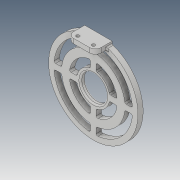
# Autodesk Inventor part: backSideThrusterCover
Saved by Autodesk Inventor 2018 (Build 220112000, 112)
## iProperties
Created: 2020-02-23
Part Number: backSideThrusterCover
Material: Generic
Document SubType Name: Modeling
Designer: anirudh
Density: 1 g/cm^3
Appearance: Default
Author: anirudh
Autodesk Inventor part; units mm, degrees
ref_plane "YZ Plane" through (0, 0, 0) normal (1, 0, 0) x (0, 1, 0)
ref_plane "XZ Plane" through (0, 0, 0) normal (0, 1, 0) x (-1, 0, 0)
ref_plane "XY Plane" through (0, 0, 0) normal (0, 0, 1) x (1, 0, 0)
sketch "Sketch1" plane through (0, 0, 0) normal (0, 0, 1) x (1, 0, 0)
  line L0 (3, 0) -> (-3, 0)
  line L1 (0, 0) -> (13.85, 0)
  line L2 (14.85, -3.0647) -> (14.85, -1)
  line L3 (14.85, -3.0647) -> (14.85, -1)
  line L4 (0, 0) -> (-13.85, 0)
  line L5 (13.85, 0) -> (-13.85, 0)
  line L6 (-14.85, -3.0647) -> (-14.85, -1)
  line L7 (-14.85, -3.0647) -> (-14.85, -1)
  arc A0 (47.8846, -42.8653) -> (14.85, -3.0647) centre (0, -49) ccw
  arc A1 (-14.85, -3.0647) -> (14.85, -3.0647) centre (0, -49) ccw
  circle A2 centre (0, -49) radius 13.97
  arc A3 (3.175, -66.4942) -> (17.4942, -52.175) centre (0, -49) ccw
  arc A4 (-17.4942, -52.175) -> (-3.175, -66.4942) centre (0, -49) ccw
  arc A5 (17.4942, -45.825) -> (3.175, -31.5058) centre (0, -49) ccw
  arc A6 (-3.175, -31.5058) -> (-17.4942, -45.825) centre (0, -49) ccw
  line L8 (-17.4942, -52.175) -> (-25.8407, -52.175)
  line L9 (-34.1427, -52.175) -> (-42.4264, -52.175)
  line L10 (-3.175, -66.4942) -> (-3.175, -74.8407)
  line L11 (-3.175, -83.1427) -> (-3.175, -91.4264)
  arc A7 (-25.8407, -52.175) -> (-3.175, -74.8407) centre (0, -49) ccw
  line L12 (3.175, -66.4942) -> (3.175, -74.8407)
  line L13 (3.175, -83.1427) -> (3.175, -91.4264)
  line L14 (17.4942, -52.175) -> (25.8407, -52.175)
  line L15 (34.1427, -52.175) -> (42.4264, -52.175)
  arc A8 (3.175, -74.8407) -> (25.8407, -52.175) centre (0, -49) ccw
  line L16 (17.4942, -45.825) -> (25.8407, -45.825)
  line L17 (34.1427, -45.825) -> (42.4264, -45.825)
  line L18 (3.175, -31.5058) -> (3.175, -23.1593)
  line L19 (3.175, -14.8573) -> (3.175, -6.5736)
  arc A9 (25.8407, -45.825) -> (3.175, -23.1593) centre (0, -49) ccw
  arc A10 (-3.175, -23.1593) -> (-25.8407, -45.825) centre (0, -49) ccw
  line L20 (-3.175, -31.5058) -> (-3.175, -23.1593)
  line L21 (-3.175, -14.8573) -> (-3.175, -6.5736)
  line L22 (-17.4942, -45.825) -> (-25.8407, -45.825)
  line L23 (-34.1427, -45.825) -> (-42.4264, -45.825)
  arc A11 (-42.4264, -52.175) -> (-3.175, -91.4264) centre (0, -49) ccw
  arc A12 (-34.1427, -52.175) -> (-3.175, -83.1427) centre (0, -49) ccw
  arc A13 (3.175, -91.4264) -> (42.4264, -52.175) centre (0, -49) ccw
  arc A14 (3.175, -83.1427) -> (34.1427, -52.175) centre (0, -49) ccw
  arc A15 (34.1427, -45.825) -> (3.175, -14.8573) centre (0, -49) ccw
  arc A16 (-3.175, -14.8573) -> (-34.1427, -45.825) centre (0, -49) ccw
  arc A17 (42.4264, -45.825) -> (3.175, -6.5736) centre (0, -49) ccw
  arc A18 (-3.175, -6.5736) -> (-42.4264, -45.825) centre (0, -49) ccw
  line L24 (-14.85, -1) -> (-14.85, 0)
  line L25 (-14.85, 0) -> (-13.85, 0)
  line L26 (14.85, -1) -> (14.85, 0)
  line L27 (14.85, 0) -> (13.85, 0)
  point P0 (0, 0)
  point P1 (0, -49)
  point P2 (-16.85, -4.0995)
  constraints: 57 end point, 36 point on circle, 19 centre point, 8 parallel, 6 coincident, 6 perpendicular, 5 vertical, 2 horizontal, 1 collinear, 1 midpoint
extrude "Extrusion1" add sketch "Sketch1" along normal blind 5.588
fillet "Fillet1" radius 1.5875 34 edges at (14.85, -3.0647, 2.794) (-14.85, -3.0647, 2.794) (3.175, -6.5736, 2.794) (3.175, -14.8573, 2.794) (3.175, -23.1593, 2.794) (3.175, -31.5058, 2.794) (17.4942, -45.825, 2.794) (25.8407, -45.825, 2.794) (34.1427, -45.825, 2.794) (42.4264, -45.825, 2.794) (-3.175, -66.4942, 2.794) (-3.175, -74.8407, 2.794) (-3.175, -83.1427, 2.794) (-3.175, -91.4264, 2.794) (3.175, -91.4264, 2.794) (3.175, -83.1427, 2.794) (3.175, -74.8407, 2.794) (3.175, -66.4942, 2.794) (17.4942, -52.175, 2.794) (25.8407, -52.175, 2.794) (34.1427, -52.175, 2.794) (42.4264, -52.175, 2.794) (-42.4264, -52.175, 2.794) (-34.1427, -52.175, 2.794) (-25.8407, -52.175, 2.794) (-17.4942, -52.175, 2.794) (-17.4942, -45.825, 2.794) (-25.8407, -45.825, 2.794) (-34.1427, -45.825, 2.794) (-42.4264, -45.825, 2.794) (-3.175, -31.5058, 2.794) (-3.175, -23.1593, 2.794) (-3.175, -14.8573, 2.794) (-3.175, -6.5736, 2.794)
fillet "Fillet2" radius 1.5875 2 edges at (-13.97, -49, 5.588) (-13.97, -49, 0)
sketch "Sketch3" plane through (0, 0, 5.588) normal (0, 0, 1) x (1, 0, 0)
  line L0 (14.85, 0) -> (-14.85, 0) projected
  line L1 (-14.85, 0) -> (14.85, 0)
  line L2 (14.85, 0) -> (14.85, -5.08)
  line L3 (14.85, -5.08) -> (-14.85, -5.08)
  line L4 (-14.85, -5.08) -> (-14.85, 0)
  point P0 (0, 0)
  dimension "d16" = 5.08
  constraints: 8 end point, 2 parallel, 1 horizontal, 1 perpendicular
  measures "d16" distance of L1.end L2.end
extrude "Extrusion2" add sketch "Sketch3" along normal blind 12.7
fillet "Fillet3" radius 6.35 2 edges at (-14.85, -2.54, 18.288) (14.85, -2.54, 18.288)
fillet "Fillet4" radius 1.5875 3 edges at (-14.85, -3.5019, 5.588) (14.85, -3.5019, 5.588) (0, -5.08, 5.588)
sketch "Sketch4" plane through (-8.5, -5.08, 18.288) normal (0, -1, 0) x (1, 0, 0)
  line L0 (17, 0) -> (0, 0) projected
  circle A0 centre (0, -4.445) radius 1.75
  circle A1 centre (17, -4.445) radius 1.75
  point P0 (8.5, -18.288)
  dimension "d22" = 3.5
  dimension "d23" = 3.5
  constraints: 2 centre point
  measures "d22" diameter of A0
  measures "d23" diameter of A1
extrude "Extrusion3" cut sketch "Sketch4" against normal blind 10.16
body "Solid1"
